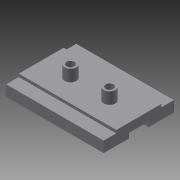
# Autodesk Inventor part: sliding piece
Saved by Autodesk Inventor 2015 SP1 (Build 190203100, 203)
## iProperties
Created: 2015-01-14
Part Number: sliding piece
Material: Generic
Document SubType Name: Modeling
Designer: Jarod
Density: 1 g/cm^3
Appearance: Default
Author: Jarod
Autodesk Inventor part; units mm, degrees
ref_plane "YZ Plane" through (0, 0, 0) normal (1, 0, 0) x (0, 1, 0)
ref_plane "XZ Plane" through (0, 0, 0) normal (0, 1, 0) x (-1, 0, 0)
ref_plane "XY Plane" through (0, 0, 0) normal (0, 0, 1) x (1, 0, 0)
sketch "Sketch1" plane through (0, 0, 0) normal (1, 0, 0) x (0, 1, 0)
  line L0 (166.4905, 202.3696) -> (166.4905, 162.3646) projected
  line L1 (166.4905, 162.3646) -> (175.9901, 162.3646) projected
  line L2 (175.9901, 162.3646) -> (175.9901, 169.8576) projected
  line L3 (175.9901, 169.8576) -> (174.4915, 169.8576) projected
  line L4 (174.4915, 169.8576) -> (174.4915, 164.3712) projected
  line L5 (174.4915, 164.3712) -> (168.9797, 164.3712) projected
  line L6 (168.9797, 164.3712) -> (168.9797, 177.376) projected
  line L7 (168.9797, 177.376) -> (171.4689, 177.376) projected
  line L8 (171.4689, 177.376) -> (170.4783, 178.3666) projected
  line L9 (170.4783, 178.3666) -> (170.4783, 186.3676) projected
  line L10 (170.4783, 186.3676) -> (171.4689, 187.3582) projected
  line L11 (171.4689, 187.3582) -> (168.9797, 187.3582) projected
  line L12 (168.9797, 187.3582) -> (168.9797, 200.363) projected
  line L13 (168.9797, 200.363) -> (174.4915, 200.363) projected
  line L14 (174.4915, 200.363) -> (174.4915, 194.8766) projected
  line L15 (174.4915, 194.8766) -> (175.9901, 194.8766) projected
  line L16 (175.9901, 194.8766) -> (175.9901, 202.3696) projected
  line L17 (175.9901, 202.3696) -> (166.4905, 202.3696) projected
  line L18 (174.4915, 200.363) -> (174.4915, 193.886)
  line L19 (174.4915, 200.363) -> (180.9685, 200.363) construction
  line L20 (174.4915, 200.363) -> (168.9797, 200.363)
  line L21 (168.9797, 200.363) -> (168.9797, 187.3582)
  line L22 (168.9797, 187.3582) -> (171.4689, 187.3582)
  line L23 (171.4689, 187.3582) -> (171.4689, 177.376)
  line L24 (171.4689, 177.376) -> (168.9797, 177.376)
  line L25 (168.9797, 177.376) -> (168.9797, 164.3712)
  line L26 (168.9797, 164.3712) -> (174.4915, 164.3712)
  line L27 (174.4915, 164.3712) -> (174.4915, 170.8482)
  line L28 (174.4915, 164.3712) -> (180.9685, 164.3712) construction
  line L29 (174.4915, 193.886) -> (175.9901, 193.886)
  line L30 (174.4915, 170.8482) -> (175.9901, 170.8482)
  line L31 (175.9901, 193.886) -> (175.9901, 170.8482)
  point P0 (0, 0)
  dimension "d0" = 6.477
  dimension "d1" = 90
  dimension "d2" = 6.477
  dimension "d3" = 90
  constraints: 28 end point, 5 perpendicular, 4 collinear, 4 horizontal, 3 vertical
  measures "d0" distance of L13.end L18.end
  measures "d1" angle of L18 L19
  measures "d2" distance of L4.end L27.end
  measures "d3" angle of L28 L27
extrude "Extrusion1" add sketch "Sketch1" along normal blind 50.038 contours L18 L29 L31 L30 L27 L4 L5 L6 L7 L23 L11 L12 L13 L14
sketch "Sketch2" plane through (0, 175.9901, 193.886) normal (0, 1, 0) x (1, 0, 0)
  line L0 (0, 23.0378) -> (0, 0) projected
  line L1 (0, 0) -> (50.038, 0) projected
  line L2 (50.038, 23.0378) -> (50.038, 0) projected
  line L3 (0, 23.0378) -> (50.038, 23.0378) projected
  circle A0 centre (15.0114, 11.5316) radius 2.9972
  circle A1 centre (35.0266, 11.5316) radius 2.9972
  circle A2 centre (15.0114, 11.5316) radius 1.9939
  circle A3 centre (35.0266, 11.5316) radius 1.9939
  point P0 (0, 193.886)
  dimension "d6" = 5.9944
  dimension "d7" = 5.9944
  dimension "d8" = 15.0114
  dimension "d9" = 15.0114
  dimension "d10" = 11.5316
  dimension "d11" = 11.5316
  dimension "d12" = 3.9878
  dimension "d13" = 3.9878
  constraints: 4 centre point, 2 coincident
  measures "d6" diameter of A0
  measures "d7" diameter of A1
  measures "d8" distance from line of A0.centre L0
  measures "d9" distance from line of L2 A1.centre
  measures "d10" distance from line of L1 A0.centre
  measures "d11" distance from line of L1 A1.centre
  measures "d12" diameter of A2
  measures "d13" diameter of A3
extrude "Extrusion2" add sketch "Sketch2" along normal blind 5.9944 contours A0 | A1
body "Solid1"
